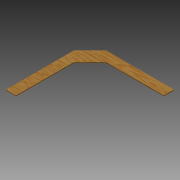
# Autodesk Inventor part: leg
Saved by Autodesk Inventor 2013 (Build 170138000, 138)
## iProperties
Created: 2014-10-20
Part Number: leg
Material: Plywood, Finish
Document SubType Name: Modeling
Designer: Masta
Density: 1 g/cm^3
Author: Masta
Autodesk Inventor part; units mm, degrees
ref_plane "YZ Plane" through (0, 0, 0) normal (1, 0, 0) x (0, 1, 0)
ref_plane "XZ Plane" through (0, 0, 0) normal (0, 1, 0) x (-1, 0, 0)
ref_plane "XY Plane" through (0, 0, 0) normal (0, 0, 1) x (1, 0, 0)
sketch "Sketch1" plane through (0, 0, 0) normal (0, 0, 1) x (1, 0, 0)
  line L0 (0, 0) -> (400, 0)
  line L1 (400, 0) -> (400, 70.7107)
  line L2 (400, 70.7107) -> (-70.7107, 70.7107)
  line L3 (-70.7107, 70.7107) -> (0, 0) construction
  line L4 (0, 0) -> (-56.5685, -56.5685)
  line L5 (-56.5685, -56.5685) -> (-127.2792, 14.1421)
  line L6 (-127.2792, 14.1421) -> (-70.7107, 70.7107)
  dimension "d0" = 400
  dimension "d2" = 135
  dimension "d3" = 80
  dimension "d6" = 100
  constraints: 14 end point, 3 perpendicular, 2 parallel, 1 horizontal
  measures "d0" distance of L0.start L0.end
  measures "d2" angle of L0 L3
  measures "d3" distance of L0.start L4.end
  measures "d6" distance of L4.end L5.end
extrude "Extrusion1" add sketch "Sketch1" along normal blind 5
mirror "Mirror1" about plane through (-127.2792, 14.1421, 0) normal (-0.7071068, -0.7071068, 0)
body "Solid1"
